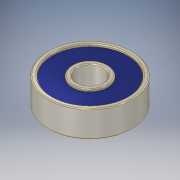
# Autodesk Inventor part: Подшипник 626Z
Saved by Autodesk Inventor 2019 (Build 230136000, 136)
## iProperties
Created: 2019-07-15
Part Number: Подшипник 626Z
Material: Титан
Document SubType Name: Modeling
Designer: user
Density: 4.51 g/cm^3
Appearance: Титан
Description: Подшипник 626Z
Mass: 6.08186 g
Surface Area: 10.2348 cm^2
Volume: 1.34853 cm^3
Author: user
Autodesk Inventor part; units mm, degrees
ref_plane "YZ Plane" through (0, 0, 0) normal (1, 0, 0) x (0, 1, 0)
ref_plane "XZ Plane" through (0, 0, 0) normal (0, 1, 0) x (-1, 0, 0)
ref_plane "XY Plane" through (0, 0, 0) normal (0, 0, 1) x (1, 0, 0)
sketch "Эскиз1" plane through (0, 0, 0) normal (0, 1, 0) x (-1, 0, 0)
  circle A0 centre (0, 0) radius 9.5
  circle A1 centre (0, 0) radius 3
  dimension "d0" = 19
  dimension "d1" = 6
  constraints: 2 centre point, 2 coincident
  measures "d0" diameter of A0
  measures "d1" diameter of A1
extrude "Выдавливание1" add sketch "Эскиз1" along normal blind 6
sketch "Эскиз2" plane through (0, 6, 0) normal (0, 1, 0) x (1, 0, 0)
  circle A0 centre (0, 0) radius 4
  circle A1 centre (0, 0) radius 8.5
  circle A2 centre (0, 0) radius 9.5 projected
  circle A3 centre (0, 0) radius 3 projected
  dimension "d4" = 1
  dimension "d5" = 1
  constraints: 2 centre point, 2 coincident
  measures "d4" radial gap between concentric circles of A1 A2
  measures "d5" radial gap between concentric circles of A3 A0
extrude "Выдавливание2" cut sketch "Эскиз2" against normal blind 0.5 contours A1
sketch "Эскиз3" plane through (0, 0, 0) normal (0, -1, 0) x (1, 0, 0)
  circle A0 centre (0, 0) radius 4 projected
  circle A1 centre (0, 0) radius 8.5 projected
extrude "Выдавливание3" cut sketch "Эскиз3" against normal blind 0.5
chamfer "Фаска1" distance 0.2 angle 45 8 edges at (-4, 0, 0) (3, 0, 0) (-8.5, 0, 0) (9.5, 0, 0) (9.5, 6, 0) (-8.5, 6, 0) (-4, 6, 0) (3, 6, 0)
